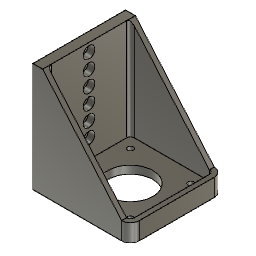
NEMA 17 Motor Mount (Autodesk Fusion 360 design; units mm, degrees)
Autodesk Fusion 360 part; units mm, degrees
sketch "Sketch7" plane through (0, 0, 0) normal (0, 0, 1) x (1, 0, 0)
  line L0 (19.25, -21.25) -> (-21.25, -21.25)
  line L1 (-21.25, -21.25) -> (-21.25, 21.25)
  line L2 (-21.25, 21.25) -> (19.25, 21.25)
  line L3 (21.25, 19.25) -> (21.25, -19.25)
  line L4 (21.25, -21.25) -> (-21.25, 21.25) construction
  line L5 (-21.25, -21.25) -> (21.25, 21.25) construction
  arc A0 (21.25, 19.25) -> (19.25, 21.25) centre (19.25, 19.25) ccw
  arc A1 (19.25, -21.25) -> (21.25, -19.25) centre (19.25, -19.25) ccw
  line L6 (19.25, -23.75) -> (-23.75, -23.75)
  line L7 (-23.75, 23.75) -> (19.25, 23.75)
  arc A2 (23.75, 19.25) -> (19.25, 23.75) centre (19.25, 19.25) ccw
  line L8 (23.75, 19.25) -> (23.75, -19.25)
  arc A3 (19.25, -23.75) -> (23.75, -19.25) centre (19.25, -19.25) ccw
  line L9 (-23.75, 23.75) -> (-26.25, 23.75)
  line L10 (-26.25, 23.75) -> (-26.25, -23.75)
  line L11 (-26.25, -23.75) -> (-23.75, -23.75)
  line L12 (-21.25, -21.25) -> (-21.25, -23.75)
  line L13 (-21.25, 21.25) -> (-21.25, 23.75)
  circle A4 centre (0, 0) radius 11.5
  dimension "d45" = 42.5
  dimension "d46" = 42.5
  dimension "d48" = 2
  dimension "d50" = 47.5
  dimension "d51" = 23
  constraint horizontal L0
  constraint perpendicular L0 L1
  constraint parallel L0 L2
  constraint parallel L1 L3
  constraint coincident L4 A4.centre
  constraint coincident L5 A4.centre
  constraint coincident A4.centre origin
  constraint coincident L5.end L2
  constraint coincident L5.end L3
  constraint tangent L2 A0
  constraint tangent L3 A0
  constraint coincident L4.start L3
  constraint coincident L4.start L0
  constraint tangent L3 A1
  constraint tangent L0 A1
  constraint equal A0 A1
  constraint perpendicular L9 L10
  constraint coincident L6 L12.end
  constraint perpendicular L6 L12
  constraint coincident L7 L13.end
  constraint perpendicular L7 L13
  constraint parallel L0 L6
  constraint parallel L2 L7
  constraint concentric A0 A2
  constraint parallel L3 L8
  constraint concentric A1 A3
  constraint tangent L7 A2
  constraint tangent L8 A3
  constraint tangent A2 L8
  constraint tangent L6 A3
  measures "d45" distance of L1.end L5.end
  measures "d46" distance of L0.end L1.end
  measures "d48" radius of A0
  measures "d50" distance of L9.end L10.end
  measures "d51" diameter of A4
extrude "Extrude8" add sketch "Sketch7" along normal blind 4 contours L0 L1 L2 L3 A0 A1 makes body 1
extrude "Extrude9" add sketch "Sketch7" along normal blind 9 contours L0 L2 L3 A0 A1 L6 L7 A2 L8 A3 L12 L13 bodies 1
extrude "Extrude10" add sketch "Sketch7" along normal blind 56 contours L1 L6 L7 L9 L10 L11 L12 L13 bodies 1
sketch "Sketch8" plane through (0, -23.75, 0) normal (0, -1, 0) x (1, 0, 0)
  line L0 (-26.25, 0) -> (19.25, 0)
  line L1 (19.25, 0) -> (19.25, 9)
  line L2 (19.25, 9) -> (-21.25, 9)
  line L3 (-21.25, 9) -> (-21.25, 56)
  line L4 (-21.25, 56) -> (-26.25, 56)
  line L5 (-26.25, 56) -> (-26.25, 0)
  line L6 (19.25, 9) -> (-21.25, 56)
  constraint coincident L1.end L2.start
  constraint coincident L3.end L4.start
extrude "Extrude11" add sketch "Sketch8" against normal blind 2.5 contours L2 L3 L6 bodies 1
fillet "Fillet2" radius 2 1 edges at (-21.25, -21.25, 30) on bodies 1
mirror "Mirror4" about plane through (0, 0, 0) normal (0, 1, 0) of "Extrude11", "Fillet2"
sketch "Sketch9" plane through (0, 0, 4) normal (0, 0, 1) x (-1, 0, 0)
  circle A0 centre (0, 0) radius 11.5
  arc A1 (19.25, -21.25) -> (21.25, -19.25) centre (19.25, -19.25) ccw
  line L0 (21.25, -19.25) -> (21.25, 19.25)
  arc A2 (21.25, 19.25) -> (19.25, 21.25) centre (19.25, 19.25) ccw
  line L1 (19.25, 21.25) -> (-19.25, 21.25)
  arc A3 (-19.25, 21.25) -> (-21.25, 19.25) centre (-19.25, 19.25) ccw
  line L2 (-21.25, 19.25) -> (-21.25, -19.25)
  arc A4 (-21.25, -19.25) -> (-19.25, -21.25) centre (-19.25, -19.25) ccw
  line L3 (-19.25, -21.25) -> (19.25, -21.25)
  line L4 (0, 0) -> (15.5, 0) construction
  line L5 (15.5, 0) -> (15.5, -15.5) construction
  dimension "d64" = 15.5
  dimension "d65" = 15.5
  constraint coincident A0.centre L4.start
  constraint horizontal L4
  constraint perpendicular L4 L5
  measures "d64" distance of A0.centre L4.end
  measures "d65" distance of L4.end L5.end
hole "Hole2" at (-15.5, 15.5, 4) direction (0, 0, -1) diameter 3 end through all bodies 1
mirror "Mirror5" about plane through (0, 0, 0) normal (1, 0, 0) of "Hole2"
mirror "Mirror6" about plane through (0, 0, 0) normal (0, 1, 0) of "Hole2", "Mirror5"
sketch "Sketch10" plane through (-21.25, 0, 0) normal (1, 0, 0) x (0, 1, 0)
  line L0 (19.25, 4) -> (19.25, 56)
  line L1 (19.25, 56) -> (-19.25, 56)
  line L2 (-19.25, 56) -> (-19.25, 4)
  line L3 (-19.25, 4) -> (19.25, 4)
  line L4 (-19.25, 9) -> (19.25, 9) construction
  line L5 (0, 56) -> (0, 9) construction
  circle A0 centre (0, 51.5943) radius 3
  circle A1 centre (0, 43.9943) radius 3
  circle A2 centre (0, 36.3943) radius 3
  circle A3 centre (0, 28.7943) radius 3
  circle A4 centre (0, 21.1943) radius 3
  circle A5 centre (0, 13.5943) radius 3
  circle A6 centre (0, 51.5943) radius 1.5
  circle A7 centre (0, 43.9943) radius 1.5
  circle A8 centre (0, 36.3943) radius 1.5
  circle A9 centre (0, 28.7943) radius 1.5
  circle A10 centre (0, 21.1943) radius 1.5
  circle A11 centre (0, 13.5943) radius 1.5
  dimension "d73" = 6
  dimension "d76" = 0
  dimension "d77" = -38
  dimension "d78" = 3
  dimension "d81" = 0
  dimension "d82" = -38
  constraint midpoint L1 L5.start
  constraint midpoint L4 L5.end
  constraint coincident L5 A0.centre
  constraint concentric A0 A6
  measures "d73" diameter of A0
  measures "d78" diameter of A6
extrude "Extrude12" cut sketch "Sketch10" against normal through all contours A6 | A7 | A8 | A9 | A10 | A11 bodies 1
extrude "Extrude13" cut sketch "Sketch10" against normal blind 3.35 contours A0 | A1 | A2 | A3 | A4 | A5 bodies 1
copy_body "Body->Comp1" bodies 1 removing the originals makes body 2 in component "Motor Mount"
component "Motor Mount" placed x (1, 0, 0) y (0, 1, 0) z (0, 0, 1) at (0, 0, 0)
equation "d64 = ( 31 / 2 ) * 1 mm"
equation "d65 = ( 31 / 2 ) * 1 mm"
